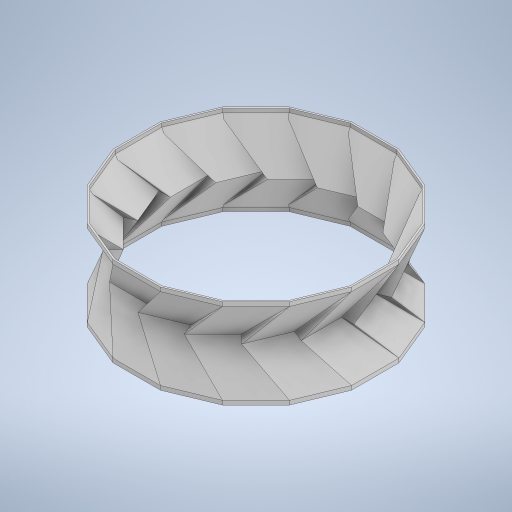
# Autodesk Inventor part: OV-PAM_n_16_standard_1F
Saved by Autodesk Inventor 2024 (Build 280153000, 153)
## iProperties
Created: 2023-08-31
Part Number: OV-PAM_n_16_standard_1F
Material: 일반
Document SubType Name: Modeling
Designer: jsw
Density: 1 g/cm^3
Appearance: 기본값
Author: jsw
Autodesk Inventor part; units mm, degrees
ref_plane "YZ Plane" through (0, 0, 0) normal (1, 0, 0) x (0, 1, 0)
sketch "스케치1" plane through (0, 0, 0) normal (0, 1, 0) x (-1, 0, 0)
  line L0 (-6.8822, 34.5992) -> (6.8822, 34.5992)
  line L1 (6.8822, 34.5992) -> (19.5989, 29.3318)
  line L2 (19.5989, 29.3318) -> (29.3318, 19.5989)
  line L3 (29.3318, 19.5989) -> (34.5992, 6.8822)
  line L4 (34.5992, 6.8822) -> (34.5992, -6.8822)
  line L5 (34.5992, -6.8822) -> (29.3318, -19.5989)
  line L6 (29.3318, -19.5989) -> (19.5989, -29.3318)
  line L7 (19.5989, -29.3318) -> (6.8822, -34.5992)
  line L8 (6.8822, -34.5992) -> (-6.8822, -34.5992)
  line L9 (-6.8822, -34.5992) -> (-19.5989, -29.3318)
  line L10 (-19.5989, -29.3318) -> (-29.3318, -19.5989)
  line L11 (-29.3318, -19.5989) -> (-34.5992, -6.8822)
  line L12 (-34.5992, -6.8822) -> (-34.5992, 6.8822)
  line L13 (-34.5992, 6.8822) -> (-29.3318, 19.5989)
  line L14 (-29.3318, 19.5989) -> (-19.5989, 29.3318)
  line L15 (-19.5989, 29.3318) -> (-6.8822, 34.5992)
  line L16 (7.0015, -35.1992) -> (-7.0015, -35.1992)
  line L17 (-7.0015, -35.1992) -> (-19.9387, -29.8404)
  line L18 (-19.9387, -29.8404) -> (-29.8404, -19.9387)
  line L19 (-29.8404, -19.9387) -> (-35.1992, -7.0015)
  line L20 (-35.1992, -7.0015) -> (-35.1992, 7.0015)
  line L21 (-35.1992, 7.0015) -> (-29.8404, 19.9387)
  line L22 (-29.8404, 19.9387) -> (-19.9387, 29.8404)
  line L23 (-19.9387, 29.8404) -> (-7.0015, 35.1992)
  line L24 (-7.0015, 35.1992) -> (7.0015, 35.1992)
  line L25 (7.0015, 35.1992) -> (19.9387, 29.8404)
  line L26 (19.9387, 29.8404) -> (29.8404, 19.9387)
  line L27 (29.8404, 19.9387) -> (35.1992, 7.0015)
  line L28 (35.1992, 7.0015) -> (35.1992, -7.0015)
  line L29 (35.1992, -7.0015) -> (29.8404, -19.9387)
  line L30 (29.8404, -19.9387) -> (19.9387, -29.8404)
  line L31 (19.9387, -29.8404) -> (7.0015, -35.1992)
  point P0 (0, 0)
  point P1 (0, 0)
  point P2 (0, 0)
  dimension "d0" = 70.554
  dimension "d1" = 0.6
  constraints: 64 end point, 2 coincident, 2 horizontal, 66 other
  measures "d0" distance of L11.end L3.end
  measures "d1" distance between parallel lines of L4 L28
extrude "돌출1" add sketch "스케치1" along normal blind 12 contours L0 L1 L2 L3 L4 L5 L6 L7 L8 L9 L10 L11 L12 L13 L14 L15 | L16 L17 L18 L19 L20 L21 L22 L23 L24 L25 L26 L27 L28 L29 L30 L31
ref_plane "작업 평면1" through (29.8404, 0, 19.9387) normal (-0.8001031, -0.5, -0.3314136) x (0.3826834, 0, -0.9238795)
sketch "스케치2" plane through (35.1992, 0, 7.0015) normal (0.9238795, 0, 0.3826834) x (0.3826834, 0, -0.9238795)
  line L0 (-14.0031, 0) -> (0, 0) projected
  line L1 (0, 0) -> (0, 12) projected
  line L2 (-14.0031, 12) -> (0, 12) projected
  line L3 (-14.0031, 0) -> (-14.0031, 12) projected
  line L4 (-14.0031, 12) -> (-34.7877, 12)
  line L5 (-34.7877, 12) -> (-14.0031, 0)
  line L6 (0, 0) -> (-10, 12)
  point P0 (-7.0015, 0)
  dimension "d5" = 150
  dimension "d6" = 10
  constraints: 6 end point, 1 horizontal, 1 point on line
  measures "d5" angle of L5 L0
  measures "d6" distance of L1.end L6.end
extrude "돌출2" cut sketch "스케치2" against normal up to surface contours L3 L2 L6 L0 | L5 L4 L3 surface through (29.8404, 0, 19.9387) normal (-0.8001031, -0.5, -0.3314136)
pattern_circular "원형 패턴1" count 16 over 360 about axis through (0, -10, 0) along (0, 1, 0) of "돌출2"
sketch "스케치3" plane through (0, 0, 0) normal (0, -1, 0) x (1, 0, 0)
  line L0 (-19.9387, -29.8404) -> (-29.8404, -19.9387) projected
  line L1 (-7.0015, -35.1992) -> (-19.9387, -29.8404) projected
  line L2 (7.0015, -35.1992) -> (-7.0015, -35.1992) projected
  line L3 (19.9387, -29.8404) -> (7.0015, -35.1992) projected
  line L4 (29.8404, -19.9387) -> (19.9387, -29.8404) projected
  line L5 (35.1992, -7.0015) -> (29.8404, -19.9387) projected
  line L6 (35.1992, 7.0015) -> (35.1992, -7.0015) projected
  line L7 (29.8404, 19.9387) -> (35.1992, 7.0015) projected
  line L8 (19.9387, 29.8404) -> (29.8404, 19.9387) projected
  line L9 (7.0015, 35.1992) -> (19.9387, 29.8404) projected
  line L10 (-7.0015, 35.1992) -> (7.0015, 35.1992) projected
  line L11 (-19.9387, 29.8404) -> (-7.0015, 35.1992) projected
  line L12 (-29.8404, 19.9387) -> (-19.9387, 29.8404) projected
  line L13 (-35.1992, 7.0015) -> (-29.8404, 19.9387) projected
  line L14 (-35.1992, -7.0015) -> (-35.1992, 7.0015) projected
  line L15 (-29.8404, -19.9387) -> (-35.1992, -7.0015) projected
  point P0 (0, 0)
extrude "돌출3" add sketch "스케치3" along normal blind 1.2
ref_plane "작업 평면2" through (0, 12, 0) normal (0, 1, 0) x (1, 0, 0)
mirror "미러1" about plane through (0, 12, 0) normal (0, 1, 0) of "돌출2", "원형 패턴1", "돌출3", "돌출1"
shell "쉘1" thickness 0.5 removed faces 2 at (2.3338, 25.2, 11.7331) at (2.3338, -1.2, 11.7331)
